Autodesk Inventor part; units mm, degrees
(part 2 of 2)
  line L146 (21.1828, -214.1721) -> (21.709, -214.1721)
  line L147 (25.0324, -218.9479) -> (22.2128, -218.9479)
  line L148 (22.2128, -218.9479) -> (22.2128, -218.2995)
  spline S175 degree 2 poles (22.2128, -218.2995) (22.5167, -218.0143) (23.0576, -217.4844) (23.3169, -217.1992) knots 0 0 0 1 2 2 2
  spline S176 degree 2 poles (23.3169, -217.1992) (23.8393, -216.6249) (24.221, -215.9357) (24.221, -215.5689) knots 0 0 0 1 2 2 2
  spline S177 degree 2 poles (24.221, -215.5689) (24.221, -215.3763) (24.1024, -215.0873) (23.995, -214.9947) knots 0 0 0 1 2 2 2
  spline S178 degree 2 poles (23.995, -214.9947) (23.8875, -214.902) (23.6059, -214.8094) (23.4355, -214.8094) knots 0 0 0 1 2 2 2
  spline S179 degree 2 poles (23.4355, -214.8094) (23.2725, -214.8094) (22.939, -214.8909) (22.7871, -214.9539) knots 0 0 0 1 2 2 2
  spline S180 degree 2 poles (22.7871, -214.9539) (22.6574, -215.0058) (22.4166, -215.154) (22.3425, -215.2058) knots 0 0 0 1 2 2 2
  line L149 (22.3425, -215.2058) -> (22.3092, -215.2058)
  line L150 (22.3092, -215.2058) -> (22.3092, -214.5538)
  spline S181 degree 2 poles (22.3092, -214.5538) (22.4981, -214.4611) (23.1762, -214.2796) (23.48, -214.2796) knots 0 0 0 1 2 2 2
  spline S182 degree 2 poles (23.48, -214.2796) (24.1209, -214.2796) (24.8434, -214.9576) (24.8434, -215.5356) knots 0 0 0 1 2 2 2
  spline S183 degree 2 poles (24.8434, -215.5356) (24.8434, -215.8061) (24.7174, -216.2581) (24.6063, -216.4507) knots 0 0 0 1 2 2 2
  spline S184 degree 2 poles (24.6063, -216.4507) (24.4951, -216.6508) (24.1728, -217.0435) (23.995, -217.2325) knots 0 0 0 1 2 2 2
  spline S185 degree 2 poles (23.995, -217.2325) (23.706, -217.5474) (22.9983, -218.2217) (22.7871, -218.4181) knots 0 0 0 1 2 2 2
  line L151 (22.7871, -218.4181) -> (25.0324, -218.4181)
  line L152 (25.0324, -218.4181) -> (25.0324, -218.9479)
  spline S186 degree 2 poles (28.4892, -216.6619) (28.4892, -217.892) (27.7741, -219.0443) (27.0294, -219.0443) knots 0 0 0 1 2 2 2
  spline S187 degree 2 poles (27.0294, -219.0443) (26.2736, -219.0443) (25.5659, -217.8698) (25.5659, -216.6656) knots 0 0 0 1 2 2 2
  spline S188 degree 2 poles (25.5659, -216.6656) (25.5659, -215.4281) (26.281, -214.2833) (27.0294, -214.2833) knots 0 0 0 1 2 2 2
  spline S189 degree 2 poles (27.0294, -214.2833) (27.7815, -214.2833) (28.4892, -215.4689) (28.4892, -216.6619) knots 0 0 0 1 2 2 2
  spline S190 degree 2 poles (27.7037, -218.055) (27.7926, -217.829) (27.8667, -217.1325) (27.8667, -216.6619) knots 0 0 0 1 2 2 2
  spline S191 degree 2 poles (27.8667, -216.6619) (27.8667, -216.1914) (27.7926, -215.4985) (27.7, -215.2651) knots 0 0 0 1 2 2 2
  spline S192 degree 2 poles (27.7, -215.2651) (27.6074, -215.0317) (27.285, -214.7909) (27.0294, -214.7909) knots 0 0 0 1 2 2 2
  spline S193 degree 2 poles (27.0294, -214.7909) (26.7737, -214.7909) (26.444, -215.0317) (26.3477, -215.2725) knots 0 0 0 1 2 2 2
  spline S194 degree 2 poles (26.3477, -215.2725) (26.255, -215.506) (26.1883, -216.2173) (26.1883, -216.6656) knots 0 0 0 1 2 2 2
  spline S195 degree 2 poles (26.1883, -216.6656) (26.1883, -217.1473) (26.2476, -217.792) (26.3439, -218.0439) knots 0 0 0 1 2 2 2
  spline S196 degree 2 poles (26.3439, -218.0439) (26.4329, -218.281) (26.7626, -218.5367) (27.0294, -218.5367) knots 0 0 0 1 2 2 2
  spline S197 degree 2 poles (27.0294, -218.5367) (27.2813, -218.5367) (27.6111, -218.2958) (27.7037, -218.055) knots 0 0 0 1 2 2 2
  line L153 (31.8941, -218.9479) -> (29.0745, -218.9479)
  line L154 (29.0745, -218.9479) -> (29.0745, -218.2995)
  spline S198 degree 2 poles (29.0745, -218.2995) (29.3784, -218.0143) (29.9193, -217.4844) (30.1786, -217.1992) knots 0 0 0 1 2 2 2
  spline S199 degree 2 poles (30.1786, -217.1992) (30.7011, -216.6249) (31.0827, -215.9357) (31.0827, -215.5689) knots 0 0 0 1 2 2 2
  spline S200 degree 2 poles (31.0827, -215.5689) (31.0827, -215.3763) (30.9641, -215.0873) (30.8567, -214.9947) knots 0 0 0 1 2 2 2
  spline S201 degree 2 poles (30.8567, -214.9947) (30.7492, -214.902) (30.4676, -214.8094) (30.2972, -214.8094) knots 0 0 0 1 2 2 2
  spline S202 degree 2 poles (30.2972, -214.8094) (30.1342, -214.8094) (29.8007, -214.8909) (29.6488, -214.9539) knots 0 0 0 1 2 2 2
  spline S203 degree 2 poles (29.6488, -214.9539) (29.5192, -215.0058) (29.2783, -215.154) (29.2042, -215.2058) knots 0 0 0 1 2 2 2
  line L155 (29.2042, -215.2058) -> (29.1709, -215.2058)
  line L156 (29.1709, -215.2058) -> (29.1709, -214.5538)
  spline S204 degree 2 poles (29.1709, -214.5538) (29.3598, -214.4611) (30.0379, -214.2796) (30.3417, -214.2796) knots 0 0 0 1 2 2 2
  spline S205 degree 2 poles (30.3417, -214.2796) (30.9826, -214.2796) (31.7051, -214.9576) (31.7051, -215.5356) knots 0 0 0 1 2 2 2
  spline S206 degree 2 poles (31.7051, -215.5356) (31.7051, -215.8061) (31.5791, -216.2581) (31.468, -216.4507) knots 0 0 0 1 2 2 2
  spline S207 degree 2 poles (31.468, -216.4507) (31.3568, -216.6508) (31.0345, -217.0435) (30.8567, -217.2325) knots 0 0 0 1 2 2 2
  spline S208 degree 2 poles (30.8567, -217.2325) (30.5677, -217.5474) (29.86, -218.2217) (29.6488, -218.4181) knots 0 0 0 1 2 2 2
  line L157 (29.6488, -218.4181) -> (31.8941, -218.4181)
  line L158 (31.8941, -218.4181) -> (31.8941, -218.9479)
  spline S209 degree 2 poles (35.3953, -217.4659) (35.3953, -217.8179) (35.1619, -218.4144) (34.9655, -218.6145) knots 0 0 0 1 2 2 2
  spline S210 degree 2 poles (34.9655, -218.6145) (34.7618, -218.8257) (34.2505, -219.0443) (33.943, -219.0443) knots 0 0 0 1 2 2 2
  spline S211 degree 2 poles (33.943, -219.0443) (33.6354, -219.0443) (33.1278, -218.8368) (32.9352, -218.6293) knots 0 0 0 1 2 2 2
  spline S212 degree 2 poles (32.9352, -218.6293) (32.6981, -218.3811) (32.4313, -217.5474) (32.4313, -216.9398) knots 0 0 0 1 2 2 2
  spline S213 degree 2 poles (32.4313, -216.9398) (32.4313, -216.3433) (32.6758, -215.3837) (32.9315, -215.028) knots 0 0 0 1 2 2 2
  spline S214 degree 2 poles (32.9315, -215.028) (33.1797, -214.6797) (33.9652, -214.2907) (34.4802, -214.2907) knots 0 0 0 1 2 2 2
  spline S215 degree 2 poles (34.4802, -214.2907) (34.6321, -214.2907) (34.8988, -214.3203) (34.9989, -214.3537) knots 0 0 0 1 2 2 2
  line L159 (34.9989, -214.3537) -> (34.9989, -214.9428)
  line L160 (34.9989, -214.9428) -> (34.9729, -214.9428)
  spline S216 degree 2 poles (34.9729, -214.9428) (34.8877, -214.8983) (34.5765, -214.8205) (34.3987, -214.8205) knots 0 0 0 1 2 2 2
  spline S217 degree 2 poles (34.3987, -214.8205) (33.8281, -214.8205) (33.1278, -215.5912) (33.0612, -216.347) knots 0 0 0 1 2 2 2
  spline S218 degree 2 poles (33.0612, -216.347) (33.2798, -216.1951) (33.7392, -216.0284) (34.0133, -216.0284) knots 0 0 0 1 2 2 2
  spline S219 degree 2 poles (34.0133, -216.0284) (34.2801, -216.0284) (34.6803, -216.1358) (34.8988, -216.2988) knots 0 0 0 1 2 2 2
  spline S220 degree 2 poles (34.8988, -216.2988) (35.1508, -216.4878) (35.3953, -217.0732) (35.3953, -217.4659) knots 0 0 0 1 2 2 2
  spline S221 degree 2 poles (34.7729, -217.4918) (34.7729, -217.2103) (34.6247, -216.8286) (34.4617, -216.6953) knots 0 0 0 1 2 2 2
  spline S222 degree 2 poles (34.4617, -216.6953) (34.3394, -216.5989) (34.0356, -216.536) (33.8763, -216.536) knots 0 0 0 1 2 2 2
  spline S223 degree 2 poles (33.8763, -216.536) (33.6614, -216.536) (33.2575, -216.6656) (33.0612, -216.7879) knots 0 0 0 1 2 2 2
  spline S224 degree 2 poles (33.0612, -216.7879) (33.0574, -216.8546) (33.05, -216.9806) (33.05, -217.0769) knots 0 0 0 1 2 2 2
  spline S225 degree 2 poles (33.05, -217.0769) (33.05, -217.5511) (33.2353, -218.1328) (33.3761, -218.2847) knots 0 0 0 1 2 2 2
  spline S226 degree 2 poles (33.3761, -218.2847) (33.5058, -218.4292) (33.7873, -218.5441) (33.9467, -218.5441) knots 0 0 0 1 2 2 2
  spline S227 degree 2 poles (33.9467, -218.5441) (34.3172, -218.5441) (34.7729, -218.018) (34.7729, -217.4918) knots 0 0 0 1 2 2 2
  point P0 (0, 0)
  constraints: 2 other
emboss "Emboss1" sketch "Sketch14" operation cut depth 2.54 direction (-1, 0, 0)
sketch "Sketch16" plane through (5.08, 0, 0) normal (1, 0, 0) x (0, 0, -1)
  line L0 (-43.0067, -86.6362) -> (38.2733, -86.6362)
  line L1 (38.2733, -86.6362) -> (38.2733, -90.4462)
  line L2 (38.2733, -90.4462) -> (-43.0067, -90.4462)
  line L3 (-43.0067, -90.4462) -> (-43.0067, -86.6362)
  line L4 (38.9083, -223.7962) -> (-43.6417, -223.7962) projected
  line L5 (42.0833, 28.0448) -> (42.0833, -220.6212) projected
  line L6 (-46.8167, -220.6212) -> (-46.8167, 28.0448) projected
  point P0 (0, 0)
  point P1 (38.2733, -88.5412)
  point P2 (-43.0067, -88.5412)
  dimension "d195" = 3.81
  dimension "d692" = 137.16
  dimension "d796" = 3.81
  dimension "d797" = 3.81
  constraints: 8 end point, 2 midpoint, 2 parallel, 1 horizontal, 1 perpendicular
  measures "d195" distance between parallel lines of L0 L2
  measures "d692" distance between parallel lines of L4 L0
  measures "d796" distance from line of L5 point (38.273, -88.541)
  measures "d797" distance from line of L6 point (-43.007, -88.541)
extrude "Extrusion13" add sketch "Sketch16" along normal blind 5.08
sketch "Sketch17" plane through (22.86, 33.2264, 21.4167) normal (0, 1, 0) x (1, 0, 0)
  line L0 (-6.858, 38.1) -> (0, 38.1) projected
  line L1 (-0.0061, 38.1) -> (0.0392, 38.1)
  line L2 (0, 65.5066) -> (0, -27.4066) projected
  line L3 (0, 35.5801) -> (0, 35.5243)
  line L4 (5, -24.2316) -> (5, 62.3316) projected
  line L5 (0, 38.1) -> (5, 38.1)
  line L6 (5, 38.1) -> (5, 0)
  line L7 (5, 0) -> (0, 0)
  line L8 (0, 0) -> (0, 38.1)
  point P0 (-22.86, 21.4167)
  point P1 (5, -23.8506)
  point P2 (5, 69.0626)
  point P3 (0, 0)
  point P4 (5, 38.1)
  point P5 (0, 38.1)
  point P6 (2.5, 0)
  point P7 (2.5, 38.1)
  dimension "d689" = 38.1
  constraints: 12 end point, 4 point on line, 2 horizontal, 2 midpoint, 2 parallel, 1 perpendicular
  measures "d689" distance of point (2.5, 0) point (2.5, 38.1)
extrude "Extrusion14" cut sketch "Sketch17" against normal blind 2.0066
sketch "Sketch18" plane through (0, 0, 0) normal (-1, 0, 0) x (0, 0, 1)
  arc A0 (46.2144, 33.1755) -> (48.7724, 30.6175) centre (48.0867, 32.4898) ccw projected
  circle A1 centre (48.0867, 32.4898) radius 4.5085
  arc A2 (-41.481, 33.1755) -> (-44.039, 30.6175) centre (-43.3533, 32.4898) ccw projected
  circle A3 centre (-43.3533, 32.4898) radius 4.5085
  arc A4 (-44.039, -223.194) -> (-41.481, -225.752) centre (-43.3533, -225.0662) ccw projected
  circle A5 centre (-43.3533, -225.0662) radius 4.5085
  arc A6 (46.2144, -225.752) -> (48.7724, -223.194) centre (48.0867, -225.0662) ccw projected
  circle A7 centre (48.0867, -225.0662) radius 4.5085
  point P0 (0, 0)
  dimension "d209" = 9.017
  dimension "d210" = 9.017
  dimension "d211" = 9.017
  dimension "d212" = 9.017
  constraints: 4 centre point, 4 coincident
  measures "d209" diameter of A1
  measures "d210" diameter of A3
  measures "d211" diameter of A5
  measures "d212" diameter of A7
extrude "Extrusion15" [suppressed]
sketch "Sketch19" plane through (22.86, -64.2842, -44.0899) normal (0, 0, -1) x (-1, 0, 0)
  line L0 (6.35, 0) -> (0, 0) projected
  line L1 (-5, 92.329) -> (-5, -156.337) projected
  line L2 (0, 0) -> (-5, 0)
  line L3 (-5, 0) -> (-5, 8.001)
  line L4 (-5, 8.001) -> (0, 8.001)
  line L5 (0, 8.001) -> (0, 0)
  point P0 (22.86, 64.2842)
  dimension "d216" = 5
  dimension "d219" = 8.001
  constraints: 8 end point, 2 parallel, 1 horizontal, 1 perpendicular, 1 point on line
  measures "d216" distance between parallel lines of L1 L5
  measures "d219" distance between parallel lines of L2 L4
extrude "Extrusion16" cut sketch "Sketch19" against normal blind 24.13
sketch "Sketch20" plane through (0, 0, 0) normal (-1, 0, 0) x (0, 0, 1)
  line L0 (-45.1249, 28.9592) -> (-41.5943, 28.9592)
  line L1 (-45.1249, 36.0204) -> (-41.5943, 36.0204)
  line L2 (-45.1249, 28.9592) -> (-47.1633, 32.4898)
  line L3 (-45.1249, 36.0204) -> (-47.1633, 32.4898)
  line L4 (-41.5943, 28.9592) -> (-39.5559, 32.4898)
  line L5 (-41.5943, 36.0204) -> (-39.5559, 32.4898)
  line L6 (49.8457, 36.0204) -> (51.8841, 32.4898)
  line L7 (49.8457, 28.9592) -> (51.8841, 32.4898)
  line L8 (46.3151, 28.9592) -> (49.8457, 28.9592)
  line L9 (46.3151, 36.0204) -> (49.8457, 36.0204)
  line L10 (46.3151, 36.0204) -> (44.2767, 32.4898)
  line L11 (46.3151, 28.9592) -> (44.2767, 32.4898)
  line L12 (43.6417, 31.2198) -> (-38.9083, 31.2198) projected
  line L13 (-45.2583, 37.5698) -> (49.9917, 37.5698) projected
  line L14 (53.1667, 34.3948) -> (53.1667, -226.9712) projected
  line L15 (41.2351, -73.1996) -> (44.7657, -73.1996)
  line L16 (44.7657, -73.1996) -> (46.8041, -76.7302)
  line L17 (41.2351, -73.1996) -> (39.1967, -76.7302)
  line L18 (44.7657, -80.2608) -> (46.8041, -76.7302)
  line L19 (41.2351, -80.2608) -> (39.1967, -76.7302)
  line L20 (41.2351, -80.2608) -> (44.7657, -80.2608)
  line L21 (-40.0449, -73.1996) -> (-42.0833, -76.7302)
  line L22 (-40.0449, -80.2608) -> (-42.0833, -76.7302)
  line L23 (-40.0449, -73.1996) -> (-36.5143, -73.1996)
  line L24 (-40.0449, -80.2608) -> (-36.5143, -80.2608)
  line L25 (-36.5143, -73.1996) -> (-34.4759, -76.7302)
  line L26 (-36.5143, -80.2608) -> (-34.4759, -76.7302)
  line L27 (-45.1249, -228.5968) -> (-41.5943, -228.5968)
  line L28 (-45.1249, -221.5356) -> (-41.5943, -221.5356)
  line L29 (-45.1249, -228.5968) -> (-47.1633, -225.0662)
  line L30 (-45.1249, -221.5356) -> (-47.1633, -225.0662)
  line L31 (-41.5943, -228.5968) -> (-39.5559, -225.0662)
  line L32 (-41.5943, -221.5356) -> (-39.5559, -225.0662)
  line L33 (46.3151, -228.5968) -> (49.8457, -228.5968)
  line L34 (46.3151, -221.5356) -> (49.8457, -221.5356)
  line L35 (46.3151, -228.5968) -> (44.2767, -225.0662)
  line L36 (46.3151, -221.5356) -> (44.2767, -225.0662)
  line L37 (49.8457, -228.5968) -> (51.8841, -225.0662)
  line L38 (49.8457, -221.5356) -> (51.8841, -225.0662)
  point P0 (0, 0)
  point P1 (-43.3596, 28.9592)
  point P2 (-43.3533, 32.4898)
  point P3 (48.0804, 28.9592)
  point P4 (-16.6833, 31.2198)
  point P5 (43.0004, -80.2608)
  point P6 (-38.2796, -80.2608)
  point P7 (-43.3596, -228.5968)
  point P8 (-43.3533, -225.0662)
  point P9 (48.0804, -228.5968)
  point P10 (48.0867, -225.0662)
  dimension "d366" = 7.0612
  dimension "d367" = 120
  dimension "d368" = 120
  dimension "d369" = 120
  dimension "d370" = 120
  dimension "d371" = 3.5306
  dimension "d372" = 3.5306
  dimension "d373" = 3.5306
  dimension "d374" = 3.5306
  dimension "d375" = 3.5306
  dimension "d376" = 3.5306
  dimension "d377" = 0
  dimension "d378" = 7.6074
  dimension "d383" = 7.0612
  dimension "d384" = 120
  dimension "d385" = 120
  dimension "d386" = 120
  dimension "d387" = 120
  dimension "d388" = 3.5306
  dimension "d389" = 3.5306
  dimension "d390" = 3.5306
  dimension "d391" = 3.5306
  dimension "d392" = 3.5306
  dimension "d393" = 3.5306
  dimension "d394" = 0
  dimension "d395" = 7.6074
  dimension "d731" = 7.0612
  dimension "d732" = 120
  dimension "d733" = 120
  dimension "d734" = 120
  dimension "d735" = 120
  dimension "d736" = 3.5306
  dimension "d737" = 3.5306
  dimension "d738" = 3.5306
  dimension "d739" = 3.5306
  dimension "d740" = 3.5306
  dimension "d741" = 3.5306
  dimension "d742" = 0
  dimension "d743" = 7.6074
  dimension "d748" = 7.0612
  dimension "d749" = 120
  dimension "d750" = 120
  dimension "d751" = 120
  dimension "d752" = 120
  dimension "d753" = 3.5306
  dimension "d754" = 3.5306
  dimension "d755" = 3.5306
  dimension "d756" = 3.5306
  dimension "d757" = 3.5306
  dimension "d758" = 3.5306
  dimension "d759" = 0
  dimension "d760" = 7.6074
  dimension "d798" = 7.0612
  dimension "d799" = 120
  dimension "d800" = 120
  dimension "d801" = 120
  dimension "d802" = 120
  dimension "d803" = 3.5306
  dimension "d804" = 3.5306
  dimension "d805" = 3.5306
  dimension "d806" = 3.5306
  dimension "d807" = 3.5306
  dimension "d808" = 3.5306
  dimension "d809" = 0
  constraints: 72 end point, 12 horizontal, 6 midpoint
  measures "d366" distance from line of point (-43.36, 28.959) L1
  measures "d367" angle of L0 L2
  measures "d368" angle of L1 L3
  measures "d369" angle of L4 L0
  measures "d370" angle of L5 L1
  measures "d371" distance of L0.start L4.start
  measures "d372" distance of L1.start L5.start
  measures "d373" vertical distance of L1.start L3.end
  measures "d374" vertical distance of L0.start L2.end
  measures "d375" vertical distance of L5.start L5.end
  measures "d376" vertical distance of L4.start L4.end
  measures "d377" horizontal distance of L0.start L1.start
  measures "d378" distance of L4.end L2.end
  measures "d383" distance from line of point (48.08, 28.959) L9
  measures "d384" angle of L8 L11
  measures "d385" angle of L9 L10
  measures "d386" angle of L7 L8
  measures "d387" angle of L6 L9
  measures "d388" distance of L8.start L7.start
  measures "d389" distance of L9.start L6.start
  measures "d390" vertical distance of L9.start L10.end
  measures "d391" vertical distance of L8.start L11.end
  measures "d392" vertical distance of L6.start L6.end
  measures "d393" vertical distance of L7.start L7.end
  measures "d394" horizontal distance of L8.start L9.start
  measures "d395" distance of L7.end L11.end
  measures "d731" distance from line of point (43, -80.261) L15
  measures "d732" angle of L20 L19
  measures "d733" angle of L15 L17
  measures "d734" angle of L18 L20
  measures "d735" angle of L16 L15
  measures "d736" distance of L19.start L20.end
  measures "d737" distance of L17.start L15.end
  measures "d738" vertical distance of L17.start L17.end
  measures "d739" vertical distance of L19.start L19.end
  measures "d740" vertical distance of L15.end L16.end
  measures "d741" vertical distance of L20.end L18.end
  measures "d742" horizontal distance of L19.start L17.start
  measures "d743" distance of L18.end L19.end
  measures "d748" distance from line of point (-38.28, -80.261) L23
  measures "d749" angle of L24 L22
  measures "d750" angle of L23 L21
  measures "d751" angle of L26 L24
  measures "d752" angle of L25 L23
  measures "d753" distance of L24.start L24.end
  measures "d754" distance of L23.start L25.start
  measures "d755" vertical distance of L23.start L21.end
  measures "d756" vertical distance of L24.start L22.end
  measures "d757" vertical distance of L25.start L25.end
  measures "d758" vertical distance of L24.end L26.end
  measures "d759" horizontal distance of L24.start L23.start
  measures "d760" distance of L26.end L22.end
  measures "d798" distance from line of point (-43.36, -228.597) L28
  measures "d799" angle of L27 L29
  measures "d800" angle of L28 L30
  measures "d801" angle of L31 L27
  measures "d802" angle of L32 L28
  measures "d803" distance of L27.start L31.start
  measures "d804" distance of L28.start L32.start
  measures "d805" vertical distance of L28.start L30.end
  measures "d806" vertical distance of L27.start L29.end
  measures "d807" vertical distance of L32.start L32.end
  measures "d808" vertical distance of L31.start L31.end
  measures "d809" horizontal distance of L27.start L28.start
extrude "Extrusion18" cut sketch "Sketch20" against normal blind 4
sketch "Sketch21" plane through (5.08, 0, 0) normal (1, 0, 0) x (0, 0, -1)
  line L0 (-46.8167, -220.6212) -> (-46.8167, 28.0448) projected
  line L1 (35.2253, -82.5002) -> (35.2253, -72.3775)
  line L2 (42.0833, -65.4455) -> (42.0833, -88.8822)
  circle A0 centre (38.2733, -76.7302) radius 1.9939
  line L3 (42.0833, -69.6717) -> (42.0833, -83.8957)
  line L4 (35.2282, -81.9518) -> (35.2282, -71.6157)
  line L5 (36.9596, -68.7879) -> (40.1092, -67.18)
  line L6 (41.4701, -65.8406) -> (42.0833, -64.6853)
  line L7 (36.9596, -84.7796) -> (40.1092, -86.3875)
  line L8 (41.4701, -87.7269) -> (42.0833, -88.8822)
  arc A1 (36.9596, -68.7879) -> (35.2282, -71.6157) centre (38.4032, -71.6157) ccw
  arc A2 (40.1092, -67.18) -> (41.4701, -65.8406) centre (38.6656, -64.3522) ccw
  arc A3 (35.2282, -81.9518) -> (36.9596, -84.7796) centre (38.4032, -81.9518) ccw
  arc A4 (41.4701, -87.7269) -> (40.1092, -86.3875) centre (38.6656, -89.2153) ccw
  circle A5 centre (38.2733, -76.7302) radius 1.9939 projected
  line L9 (44.0899, -222.6278) -> (44.0899, -64.2842) projected
  line L10 (42.0833, -65.4455) -> (42.0833, -64.6853)
  line L11 (-46.8167, -83.8422) -> (-46.8167, -69.6182)
  line L12 (-39.9587, -71.5622) -> (-39.9587, -81.8983)
  circle A6 centre (-43.0067, -76.7302) radius 1.9939 projected
  line L13 (-41.6901, -84.7261) -> (-44.8397, -86.334)
  line L14 (-46.1908, -87.655) -> (-46.8167, -88.8159)
  line L15 (-41.6901, -68.7344) -> (-44.8397, -67.1265)
  line L16 (-46.2239, -65.7423) -> (-46.8167, -64.5811)
  arc A7 (-44.8397, -86.334) -> (-46.1908, -87.655) centre (-43.3961, -89.1618) ccw
  arc A8 (-41.6901, -84.7261) -> (-39.9587, -81.8983) centre (-43.1337, -81.8983) ccw
  arc A9 (-39.9587, -71.5622) -> (-41.6901, -68.7344) centre (-43.1337, -71.5622) ccw
  arc A10 (-46.2239, -65.7423) -> (-44.8397, -67.1265) centre (-43.3961, -64.2987) ccw
  line L17 (-46.8167, -64.5811) -> (-46.8167, -88.8159)
  point P0 (0, 0)
  point P1 (41.0008, -66.7248)
  point P2 (41.0008, -86.8426)
  point P3 (-45.7211, -86.7839)
  point P4 (-45.7561, -66.6587)
  dimension "d766" = 6.858
  dimension "d767" = 3.9878
  dimension "d768" = 2.0396
  dimension "d769" = 2.0396
  dimension "d770" = 117.044
  dimension "d771" = 117.044
  dimension "d772" = 3.175
  dimension "d773" = 3.1496
  dimension "d774" = 3.1496
  dimension "d775" = 145
  dimension "d776" = 145
  dimension "d778" = 0
  dimension "d779" = 0
  dimension "d782" = 0
  dimension "d785" = 6.858
  dimension "d786" = 117.044
  dimension "d787" = 117.044
  dimension "d792" = 2.032
  dimension "d793" = 3.175
  dimension "d794" = 3.1496
  dimension "d795" = 3.1496
  constraints: 32 end point, 16 point on circle, 16 tangent, 12 point on line, 9 centre point, 6 equal radius, 2 parallel, 2 vertical, 1 coincident, 1 perpendicular
  measures "d766" distance between parallel lines of L2 L1
  measures "d767" diameter of A0
  measures "d768" vertical distance of point (41.001, -86.843) L8.end
  measures "d769" vertical distance of point (41.001, -66.725) L6.end
  measures "d770" angle of L5 L4
  measures "d771" angle of L4 L7
  measures "d772" radius of A1
  measures "d773" horizontal distance of L7.start L7.end
  measures "d774" horizontal distance of L5.start L5.end
  measures "d775" angle of L7 L8
  measures "d776" angle of L5 L6
  measures "d778" distance of A5.centre A0.centre
  measures "d779" distance of L8.end L2.end
  measures "d782" distance of A5.centre A0.centre
  measures "d785" distance between parallel lines of L0 L12
  measures "d786" angle of L13 L12
  measures "d787" angle of L15 L12
  measures "d792" vertical distance of point (-45.721, -86.784) L14.end
  measures "d793" radius of A7
  measures "d794" horizontal distance of L13.start L13.end
  measures "d795" horizontal distance of L15.start L15.end
extrude "Extrusion19" add sketch "Sketch21" along normal blind 22.86
sketch "Sketch22" plane through (16.08, -230.1462, -3.2973) normal (0, -1, 0) x (1, 0, 0)
  circle A0 centre (2.2292, -12.1283) radius 2.032
  line L0 (-16.08, -45.136) -> (6.78, -45.136) projected
  circle A1 centre (8.732, -12.1283) radius 2.032
  line L1 (11.78, 48.9456) -> (11.78, -37.6176) projected
  point P0 (-16.08, 3.2973)
  dimension "d445" = 4.064
  dimension "d446" = 33.0076
  dimension "d449" = 4.064
  dimension "d450" = 3.048
  constraints: 2 centre point
  measures "d445" diameter of A0
  measures "d446" distance from line of L0 A0.centre
  measures "d449" diameter of A1
  measures "d450" distance from line of L1 A1.centre
extrude "Extrusion20" cut sketch "Sketch22" against normal blind 6.35
fillet "Fillet6" radius 0.508 10 edges at (19.685, -64.2842, -48.4333) (19.685, -56.2842, -48.4333) (16.51, -60.2842, -48.4333) (15.748, -230.1462, 6.7027) (15.748, -230.1462, -3.2973) (19.431, 37.5698, -16.6833) (16.002, 37.5698, 2.3667) (19.431, 37.5698, 21.4167) (25.36, 33.2264, 21.4167) (25.36, -56.2832, -44.0899)
sketch "Sketch23" plane through (22.86, -225.8028, -3.2973) normal (0, -1, 0) x (1, 0, 0)
  line L0 (0, -37.6176) -> (0, 48.9456) projected
  line L1 (5, 48.9456) -> (5, -37.6176) projected
  line L2 (0, 10) -> (5, 10)
  line L3 (5, 10) -> (5, -0.0129)
  line L4 (5, -0.0129) -> (0, -0.0129)
  line L5 (0, -0.0129) -> (0, 10)
  point P0 (-22.86, 3.2973)
  constraints: 8 end point, 2 parallel, 1 horizontal, 1 perpendicular, 1 point on line
extrude "Extrusion21" cut sketch "Sketch23" against normal blind 6.35
sketch "Sketch24" plane through (8.636, -223.7962, -3.2973) normal (0, 1, 0) x (1, 0, 0)
  circle A0 centre (9.652, -31.318) radius 4.445
  line L0 (-3.556, 35.611) -> (-3.556, -46.939) projected
  point P0 (-8.636, -3.2973)
  point P1 (14.224, -56.464)
  dimension "d673" = 25.146
  dimension "d674" = 13.208
  dimension "d677" = 8.89
  constraints: 1 centre point
  measures "d673" vertical distance of point (14.224, -56.464) A0.centre
  measures "d674" distance from line of L0 A0.centre
  measures "d677" diameter of A0
extrude "Extrusion22" cut sketch "Sketch24" against normal blind 3.048
sketch "Sketch25" plane through (5.08, 0, 0) normal (1, 0, 0) x (0, 0, -1)
  line L0 (-46.8167, 3.2798) -> (23.2009, 3.2798)
  line L1 (14.3109, -9.4202) -> (-46.8167, -9.4202)
  line L2 (-46.8167, -9.4202) -> (-46.8167, 3.2798)
  circle A0 centre (-30.3067, -3.0702) radius 2 projected
  circle A1 centre (6.6909, -3.0702) radius 2 projected
  circle A2 centre (-11.8079, -3.0702) radius 2 projected
  line L3 (-46.8167, -220.6212) -> (-46.8167, 28.0448) projected
  line L4 (42.0833, 28.0448) -> (42.0833, -56.2832) projected
  line L5 (23.2009, 3.2798) -> (42.0833, 3.2798)
  line L6 (42.0833, 3.2798) -> (42.0833, -9.4202)
  line L7 (42.0833, -9.4202) -> (14.3109, -9.4202)
  point P0 (0, 0)
  point P1 (-11.8079, 3.2798)
  point P2 (-46.8167, -36.8286)
  point P3 (42.0833, -36.6918)
  dimension "d680" = 6.35
  dimension "d681" = 6.35
  dimension "d682" = 0
  dimension "d685" = 0
  dimension "d686" = 12.7
  constraints: 12 end point, 2 horizontal, 2 parallel, 1 midpoint, 1 perpendicular
  measures "d680" distance of point (-11.808, 3.28) A2.centre
  measures "d681" distance from line of L1 A2.centre
  measures "d682" distance between parallel lines of L3 L2
  measures "d685" distance between parallel lines of L4 L6
  measures "d686" distance between parallel lines of L7 L5
extrude "Extrusion23" add sketch "Sketch25" along normal blind 10.16
sketch "Sketch26" plane through (0, -230.1462, -45.2583) normal (0, -1, 0) x (1, 0, 0)
  line L0 (27.934, 90.805) -> (6.4997, 90.805)
  line L1 (6.4997, 90.805) -> (6.4997, 4.445)
  line L2 (6.4997, 4.445) -> (27.934, 4.445)
  line L3 (27.934, 4.445) -> (27.934, 90.805)
  line L4 (0, -3.175) -> (22.86, -3.175) projected
  line L5 (22.86, 98.425) -> (0, 98.425) projected
  point P0 (0, 45.2583)
  dimension "d832" = 7.62
  dimension "d833" = 7.62
  constraints: 8 end point, 2 parallel, 1 horizontal, 1 perpendicular
  measures "d832" distance between parallel lines of L4 L2
  measures "d833" distance between parallel lines of L5 L0
extrude "Extrusion24" cut sketch "Sketch26" against normal blind 7.62
body "Solid1"
